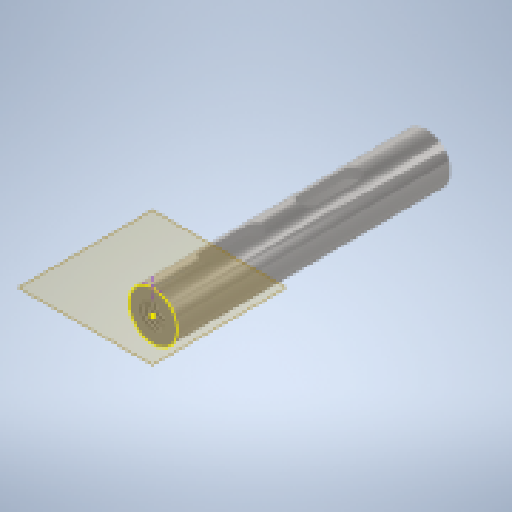
# Autodesk Inventor part: 入力軸
Saved by Autodesk Inventor 2024 (Build 280153000, 153)
## iProperties
Created: 2023-05-29
Part Number: 入力軸
Material: 鋼、炭素鋼
Document SubType Name: Modeling
Designer: yuta2
Density: 7.85 g/cm^3
Appearance: 半つや出し
Mass: 16.8186 g
Surface Area: 12.4913 cm^2
Volume: 2.1425 cm^3
Author: yuta2
Autodesk Inventor part; units mm, degrees
ref_plane "YZ Plane" through (0, 0, 0) normal (1, 0, 0) x (0, 1, 0)
ref_plane "XZ Plane" through (0, 0, 0) normal (0, 1, 0) x (-1, 0, 0)
ref_plane "XY Plane" through (0, 0, 0) normal (0, 0, 1) x (1, 0, 0)
sketch "スケッチ1" plane through (0, 0, 0) normal (1, 0, 0) x (0, 1, 0)
  line L0 (0, 0) -> (4, 0)
  line L1 (4, 0) -> (4, 4)
  line L2 (4, 4) -> (0, 4)
  line L3 (0, 4) -> (0, 0)
  line L4 (0, 0) -> (4, 0)
  line L5 (4, 0) -> (4, -55)
  line L6 (4, -55) -> (0, -55)
  line L7 (0, -55) -> (0, 0)
  line L8 (0, -55) -> (4, -55)
  line L9 (4, -55) -> (4, -59)
  line L10 (4, -59) -> (0, -59)
  line L11 (0, -59) -> (0, -55)
  point P0 (4, 0)
  dimension "d0" = 4
  dimension "d1" = 4
  dimension "d2" = 4
  dimension "d3" = 55
  dimension "d4" = 4
  dimension "d5" = 4
  constraints: 24 end point, 6 parallel, 3 horizontal, 3 perpendicular
  measures "d0" distance of L2.end L1.end
  measures "d1" distance of L1.end L0.end
  measures "d2" distance of L5.end L6.end
  measures "d3" distance of L4.end L5.end
  measures "d4" distance of L9.end L10.end
  measures "d5" distance of L8.end L9.end
revolve "回転1" add sketch "スケッチ1" angle 360 about axis through (0, 0, -55) along (0, 0, 1) contours L0 L5 L6 L7
sketch "スケッチ4" plane through (0, 0, 0) normal (0, 0, 1) x (1, 0, 0)
  circle A0 centre (0, 0) radius 4 projected
  point P0 (0, 4)
  constraints: 1 vertical alignment, 1 other
ref_plane "作業平面2" through (0, 4, 0) normal (0, 1, 0) x (-1, 0, 0)
sketch "スケッチ5" plane through (0, 4, 0) normal (0, 1, 0) x (-1, 0, 0)
  line L0 (4, -55) -> (-4, -55) projected
  line L1 (0, -55) -> (0, 0)
  line L2 (1.5, -20.5) -> (-1.5, -20.5)
  line L3 (-1.5, -20.5) -> (-1.5, -10.5)
  line L4 (-1.5, -10.5) -> (1.5, -10.5)
  line L5 (1.5, -10.5) -> (1.5, -20.5)
  line L6 (1.5, -36.5) -> (-1.5, -36.5)
  line L7 (-1.5, -36.5) -> (-1.5, -26.5)
  line L8 (-1.5, -26.5) -> (1.5, -26.5)
  line L9 (1.5, -26.5) -> (1.5, -36.5)
  arc A0 (1.5, -12) -> (-1.5, -12) centre (0, -12) ccw
  arc A1 (-1.5, -19) -> (1.5, -19) centre (0, -19) ccw
  arc A2 (1.5, -28) -> (-1.5, -28) centre (0, -28) ccw
  arc A3 (-1.5, -35) -> (1.5, -35) centre (0, -35) ccw
  dimension "d15" = 3
  dimension "d17" = 10
  dimension "d18" = 10
  dimension "d19" = 6
  dimension "d22" = 10.5
  constraints: 18 end point, 12 tangent, 10 point on line, 8 point on circle, 4 centre point, 4 parallel, 2 horizontal, 2 perpendicular, 1 midpoint, 1 vertical, 1 other
  measures "d15" distance of L6.start L6.end
  measures "d17" distance between parallel lines of L4 L2
  measures "d18" distance between parallel lines of L8 L6
  measures "d19" distance between parallel lines of L2 L8
  measures "d22" distance from line of L1.end L4
extrude "押し出し2" cut sketch "スケッチ5" against normal blind 1.8 contours A3 L7 A2 L1 | L1 A2 L9 A3 | A1 L3 A0 L1 | L1 A0 L5 A1
